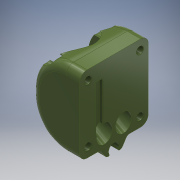
# Autodesk Inventor part: 3rd_phalanx_fingertip
Saved by Autodesk Inventor 2017 (Build 210142000, 142)
## iProperties
Created: 2017-06-28
Part Number: 3rd_phalanx_fingertip
Material: Generic
Document SubType Name: Modeling
Designer: Tomasz
Density: 1 g/cm^3
Appearance: Dark Olive
Author: Tomasz
Autodesk Inventor part; units mm, degrees
sketch "Sketch1" plane through (0, 0, 0) normal (0, 1, 0) x (-1, 0, 0)
  line L0 (0, 0) -> (1.5, 0)
  line L1 (1.5, -20) -> (0, -20)
  line L2 (0, -20) -> (0, 0)
  line L3 (1.5, 0) -> (3.5, 0)
  line L4 (12.5, -9) -> (12.5, -11)
  line L5 (3.5, -20) -> (1.5, -20)
  arc A0 (12.5, -9) -> (3.5, 0) centre (3.5, -9) ccw
  arc A1 (3.5, -20) -> (12.5, -11) centre (3.5, -11) ccw
  dimension "d0" = 20
  dimension "d4" = 9
  dimension "d5" = 12.5
  constraints: 12 end point, 4 point on circle, 4 tangent, 2 centre point, 2 horizontal, 2 parallel, 1 equal radius, 1 perpendicular, 1 point on line
  measures "d0" distance between parallel lines of L1 L0
  measures "d4" radius of A0
  measures "d5" distance between parallel lines of L4 L2
extrude "Extrusion1" add sketch "Sketch1" along normal blind 18
sketch "Sketch2" plane through (0, 0, 0) normal (1, 0, 0) x (0, 0, -1)
  line L0 (20, 0) -> (0, 0) projected
  line L1 (20, 0) -> (20, 18) projected
  line L2 (0, 18) -> (20, 18) projected
  line L3 (0, 0) -> (0, 18) projected
  line L4 (10, 0) -> (10, 18) construction
  line L5 (0, 0) -> (0, 18) projected
  line L6 (0, 9) -> (20, 9) construction
  point P0 (2.5, 2.2)
  point P1 (17.5, 2.2)
  point P2 (2.5, 15.8)
  point P3 (17.5, 15.8)
  dimension "d8" = 2.2
  dimension "d9" = 15
  constraints: 4 end point, 4 midpoint, 3 symmetric about line
  measures "d8" distance from line of L0 point (2.5, 2.2)
  measures "d9" distance of point (17.5, 2.2) point (2.5, 2.2)
hole "Hole1" at (0, 2.2, -2.5) at (0, 2.2, -17.5) at (0, 15.8, -2.5) at (0, 15.8, -17.5) direction (-1, 0, 0) diameter 1.9 end through all
ref_plane "Work Plane1" through (-2.5, 0, 0) normal (1, 0, 0) x (0, 0, -1)
sketch "Sketch3" plane through (-2.5, 0, 0) normal (1, 0, 0) x (0, 0, -1)
  spline S0 degree 2 poles (3.45, 2.2) (3.45, 0.5546) (2.025, 1.3773) (0.6, 2.2) (2.025, 3.0227) (3.45, 3.8454) (3.45, 2.2) knots 0 0 0 0.333333 0.333333 0.666667 0.666667 1 1 1 weights 1 0.5 1 0.5 1 0.5 1 projected
  spline S1 degree 2 poles (3.45, 15.8) (3.45, 14.1546) (2.025, 14.9773) (0.6, 15.8) (2.025, 16.6227) (3.45, 17.4454) (3.45, 15.8) knots 0 0 0 0.333333 0.333333 0.666667 0.666667 1 1 1 weights 1 0.5 1 0.5 1 0.5 1 projected
  spline S2 degree 2 poles (18.45, 15.8) (18.45, 14.1546) (17.025, 14.9773) (15.6, 15.8) (17.025, 16.6227) (18.45, 17.4454) (18.45, 15.8) knots 0 0 0 0.333333 0.333333 0.666667 0.666667 1 1 1 weights 1 0.5 1 0.5 1 0.5 1 projected
  spline S3 degree 2 poles (18.45, 2.2) (18.45, 0.5546) (17.025, 1.3773) (15.6, 2.2) (17.025, 3.0227) (18.45, 3.8454) (18.45, 2.2) knots 0 0 0 0.333333 0.333333 0.666667 0.666667 1 1 1 weights 1 0.5 1 0.5 1 0.5 1 projected
  circle A0 centre (2.5, 2.2) radius 0.95 projected
  circle A1 centre (2.5, 15.8) radius 0.95 projected
  circle A2 centre (17.5, 2.2) radius 0.95 projected
  circle A3 centre (17.5, 15.8) radius 0.95 projected
  circle A4 centre (2.5, 2.2) radius 1.75
  circle A5 centre (2.5, 15.8) radius 1.75
  circle A6 centre (17.5, 2.2) radius 1.75
  circle A7 centre (17.5, 15.8) radius 1.75
  point P0 (0, 0)
  dimension "d18" = 3.5
  dimension "d19" = 3.5
  dimension "d20" = 3.5
  dimension "d21" = 3.5
  constraints: 4 centre point, 4 coincident, 8 other
  measures "d18" diameter of A4
  measures "d19" diameter of A5
  measures "d20" diameter of A6
  measures "d21" diameter of A7
extrude "Extrusion2" cut sketch "Sketch3" against normal through all
sketch "Sketch4" plane through (0, 0, 0) normal (1, 0, 0) x (0, 0, -1)
  line L0 (4, 4.25) -> (16, 4.25)
  line L1 (16, 4.25) -> (16, 5.95)
  line L2 (16, 5.95) -> (4, 5.95)
  line L3 (4, 5.95) -> (4, 4.25)
  circle A0 centre (2.5, 15.8) radius 0.95 projected
  circle A1 centre (2.5, 2.2) radius 0.95 projected
  circle A2 centre (17.5, 2.2) radius 0.95 projected
  circle A3 centre (17.5, 15.8) radius 0.95 projected
  line L4 (20, 0) -> (0, 0) projected
  line L5 (20, 0) -> (20, 18) projected
  line L6 (0, 18) -> (20, 18) projected
  line L7 (0, 0) -> (0, 18) projected
  line L8 (0, 18) -> (20, 18) projected
  line L9 (20, 0) -> (0, 0) projected
  line L10 (10, 0) -> (10, 18) construction
  dimension "d25" = 12
  dimension "d26" = 1.7
  dimension "d29" = 4.25
  constraints: 10 end point, 2 midpoint, 2 parallel, 1 horizontal, 1 perpendicular, 1 other
  measures "d25" distance between parallel lines of L1 L3
  measures "d26" distance between parallel lines of L0 L2
  measures "d29" distance between parallel lines of L4 L0
extrude "Extrusion3" cut sketch "Sketch4" against normal blind 0.6 contours L3 L2 L1 L0
fillet "Fillet1" radius 2 10 edges at (-1.75, 0, -20) (-12.5, 0, -10) (-9.864, 0, -2.636) (-1.75, 0, 0) (-9.864, 0, -17.364) (-12.5, 18, -10) (-9.864, 18, -2.636) (-1.75, 18, 0) (-1.75, 18, -20) (-9.864, 18, -17.364)
ref_plane "Work Plane2" through (0, 9, 0) normal (0, -1, 0) x (1, 0, 0)
sketch "OptoForce_Offset" plane through (0, 9, 0) normal (0, -1, 0) x (1, 0, 0)
  line L0 (0, 0) -> (0, -20) projected
  line L1 (0, -10) -> (-16.7934, -10) construction
  point P0 (-10, -4)
  dimension "d30" = 10
  dimension "d31" = 6
  constraints: 2 end point, 1 horizontal, 1 midpoint
  measures "d30" distance from line of point (-10, -4) L0
  measures "d31" distance from line of point (-10, -4) L1
ref_plane "OptoForce_OffsetPlane" through (-10, 9, -4) normal (1, 0, 0) x (0, 0, -1)
sketch "OptoForce_RotationAxis" plane through (-10, 9, -4) normal (1, 0, 0) x (0, 0, -1)
  line L0 (0, 0) -> (0, 16)
  point P0 (-4, -9)
  constraints: 2 end point, 1 vertical
ref_plane "OptoForce_RotatedPlane" through (-10, 9, -4) normal (0.8660254, 0, -0.5) x (0, 1, 0)
sketch "OptoForce_SphereCenter" plane through (-10, 9, -4) normal (0.8660254, 0, -0.5) x (0, 1, 0)
  point P0 (-9, 8.4641)
  point P1 (0, 0)
ref_plane "OptoForce_OriginPlane" through (-5.6699, 9, -6.5) normal (0.8660254, 0, -0.5) x (0, 1, 0)
sketch "OptoForce_OriginSketch" plane through (-5.6699, 9, -6.5) normal (0.8660254, 0, -0.5) x (0, 1, 0)
  arc A0 (5.75, 0) -> (-5.75, 0) centre (0, 0) ccw
  line L0 (-5.75, 0) -> (-5.75, -4.25)
  line L1 (-0.5, -9.5) -> (0.5, -9.5)
  line L2 (5.75, -4.25) -> (5.75, 0)
  arc A1 (0.5, -9.5) -> (5.75, -4.25) centre (0.5, -4.25) ccw
  arc A2 (-5.75, -4.25) -> (-0.5, -9.5) centre (-0.5, -4.25) ccw
  point P0 (-9, 8.4641)
  dimension "d36" = 11.5
  dimension "d37" = 15.25
  dimension "d38" = 5.25
  constraints: 6 end point, 6 point on circle, 6 tangent, 3 centre point, 2 vertical, 1 coincident, 1 equal radius, 1 perpendicular
  measures "d36" diameter of A0
  measures "d38" radius of A1
extrude "Extrusion4" cut sketch "OptoForce_OriginSketch" against normal through all
sketch "Sketch11" plane through (-5.6699, 9, -6.5) normal (-0.8660254, 0, 0.5) x (0.5, 0, 0.8660254)
  arc A0 (0, -5.75) -> (0, 5.75) centre (0, 0) ccw projected
  line L0 (0, 5.75) -> (-4.25, 5.75) projected
  line L1 (-4.25, -5.75) -> (0, -5.75) projected
  line L2 (0, 0) -> (-14.8035, 0) construction
  line L3 (-6, -5) -> (-6, 4.6962) construction
  arc A1 (-9.5, -0.5) -> (-4.25, -5.75) centre (-4.25, -0.5) ccw projected
  arc A2 (-4.25, 5.75) -> (-9.5, 0.5) centre (-4.25, 0.5) ccw projected
  line L4 (-9.5, 0.5) -> (-9.5, -0.5) projected
  point P0 (8.4641, -9)
  point P1 (-6, -2.5)
  point P2 (-6, 2.5)
  dimension "d41" = 6
  dimension "d42" = 5
  constraints: 4 end point, 1 horizontal, 1 point on line, 1 symmetric about line, 1 vertical
  measures "d41" distance from line of L3 L2.start
  measures "d42" distance of point (-6, 2.5) point (-6, -2.5)
hole "Hole2" at (-8.6699, 6.5, -11.6962) at (-8.6699, 11.5, -11.6962) direction (0.8660254, 0, -0.5) diameter 2.4 end through all
sketch "Sketch12" plane through (-5.6699, 9, -6.5) normal (0.8660254, 0, -0.5) x (0, 1, 0)
  arc A0 (-3.5347, -5.3923) -> (-3.05, -4.9335) centre (-2.5, -6) ccw projected
  arc A1 (-3.05, -4.9335) -> (-3.6599, -5.6923) centre (-2.5, -6) ccw projected
  arc A2 (-3.5347, -5.3923) -> (-3.6599, -5.6923) centre (-2.5, -6) ccw projected
  circle A3 centre (-2.5, -6) radius 1.2 projected
  circle A4 centre (2.5, -6) radius 1.2 projected
  circle A5 centre (2.5, -6) radius 1.2 projected
  line L0 (-15, -8) -> (18.6629, -8)
  point P0 (-9, 8.4641)
  dimension "d51" = 2
  constraints: 2 end point, 1 horizontal
  measures "d51" distance from line of L0 A0.centre
ref_plane "Work Plane8" through (-9.6699, -6, -13.4282) normal (-0.5, 0, -0.8660254) x (0, 1, 0)
sketch "Sketch13" plane through (-9.6699, -6, -13.4282) normal (-0.5, 0, -0.8660254) x (0, 1, 0)
  ellipse E0 centre (12.5, 10.0111) end of major axis (13.7, 10.0111) minor radius 0.6928 (11.95, 9.3953) -> (11.4653, 9.6603) ccw projected
  line L0 (11.95, 8.7025) -> (11.95, 9.3953) projected
  ellipse E1 centre (12.5, 9.3183) end of major axis (13.7, 9.3183) minor radius 0.6928 (11.3401, 9.1406) -> (11.95, 8.7025) ccw projected
  ellipse E2 centre (12.5, 8.6077) end of major axis (12.5, 10.6862) minor radius 1.2 (11.4653, 9.6603) -> (11.3401, 9.1406) ccw projected
  line L1 (13.7, 0) -> (11.3, 0) construction
  ellipse E3 centre (17.5, 10.0111) end of major axis (18.7, 10.0111) minor radius 0.6928 projected
  line L2 (18.7, 0) -> (16.3, 0) projected
  line L3 (17.5, 0) -> (12.5, 0) construction
  line L4 (12.5, 0) -> (12.5, -4) construction
  line L5 (12.5, -4) -> (17.5, -4) construction
  line L6 (17.5, -4) -> (17.5, 0) construction
  line L7 (15, -4) -> (15, 0) construction
  arc A0 (17, -2) -> (13, -2) centre (15, -2) ccw
  line L8 (13, -2) -> (13, -6)
  line L9 (13, -6) -> (17, -6)
  line L10 (17, -6) -> (17, -2)
  point P0 (6, 1.6603)
  dimension "d53" = 4
  dimension "d54" = 4
  dimension "d55" = 2
  constraints: 16 end point, 5 midpoint, 2 horizontal, 2 parallel, 2 point on circle, 2 tangent, 2 vertical, 1 centre point, 1 perpendicular, 1 point on line, 4 other
  measures "d53" distance between parallel lines of L5 L3
  measures "d54" distance from line of L9 A0.centre
  measures "d55" radius of A0
extrude "Extrusion5" cut sketch "Sketch13" along normal through all contours L10 L9 L8 A0
ref_plane "Work Plane9" through (-4.3708, 9, -7.25) normal (0.8660254, 0, -0.5) x (0, 1, 0)
sketch "Sketch14" plane through (-4.3708, 9, -7.25) normal (0.8660254, 0, -0.5) x (0, 1, 0)
  arc A0 (-3.5347, -5.3923) -> (-3.05, -4.9335) centre (-2.5, -6) ccw projected
  arc A1 (-3.05, -4.9335) -> (-3.6599, -5.6923) centre (-2.5, -6) ccw projected
  arc A2 (-3.5347, -5.3923) -> (-3.6599, -5.6923) centre (-2.5, -6) ccw projected
  circle A3 centre (-2.5, -6) radius 1.2 projected
  circle A4 centre (2.5, -6) radius 1.2 projected
  circle A5 centre (2.5, -6) radius 1.2 projected
  circle A6 centre (-2.5, -6) radius 2.1
  circle A7 centre (2.5, -6) radius 2.1
  point P0 (-9, 8.4641)
  dimension "d59" = 4.2
  dimension "d60" = 4.2
  constraints: 2 centre point, 2 coincident
  measures "d59" diameter of A6
  measures "d60" diameter of A7
extrude "Extrusion6" cut sketch "Sketch14" along normal through all
sketch "Sketch15" plane through (0, 0, -2) normal (1, 0, 0) x (0, 0, -1)
  line L0 (-2, 2) -> (-2, 16) projected
  line L1 (-2, 9) -> (24.8317, 9) construction
  arc A0 (20.4, 9.9798) -> (18, 9) centre (19.4, 9) ccw
  line L2 (18, 2) -> (18, 16) projected
  line L3 (20.4, 11) -> (20.4, 9.9798)
  line L4 (20.4, 11) -> (18, 12.5)
  line L5 (18, 9) -> (18, 12.5)
  line L6 (18, 2) -> (18, 16) projected
  point P0 (-2, 0)
  dimension "d64" = 2.8
  dimension "d65" = 2
  dimension "d66" = 1
  dimension "d68" = 3.5
  constraints: 8 end point, 4 point on line, 3 midpoint, 2 point on circle, 1 centre point, 1 collinear, 1 horizontal, 1 parallel, 1 tangent
  measures "d64" diameter of A0
  measures "d65" distance from line of L4.start L1
  measures "d66" distance from line of L3 A0.centre
  measures "d68" distance of L5.start L4.end
extrude "Extrusion7" add sketch "Sketch15" against normal blind 3.5
fillet "Fillet2" radius 1 2 edges at (-1.75, 11, -22.4) (-1.75, 12.5, -20)
fillet "Fillet3" radius 0.2 1 edges at (-1.75, 9.9798, -22.4)
mirror "Mirror2" about plane through (0, 9, 0) normal (0, -1, 0) of "Fillet2", "Fillet3", "Extrusion7"
sketch "Sketch16" plane through (0, 16, -20) normal (0, 0, -1) x (-1, 0, 0)
  line L0 (0, -6.6) -> (0, -2.4) projected
  line L1 (0, -1.15) -> (0, 0.75) projected
  line L2 (3.5, -2.9458) -> (3.5, 0) projected
  line L3 (0, -1.15) -> (0, 0.75) projected
  line L4 (0, -1.15) -> (3.5, -1.15) construction
  line L5 (0, -2.4) -> (3.5, -2.4) construction
  line L6 (3.5, -1.775) -> (0, -1.775) construction
  line L7 (0, -2.9458) -> (0, 0) projected
  line L8 (0, -8.4) -> (0, -5.6) projected
  line L9 (0, -7) -> (8.9367, -7) construction
  point P0 (0, -16)
  point P1 (1.75, -1.775)
  point P2 (0, -8.2124)
  point P3 (0, -5.7876)
  point P4 (1.75, -12.225)
  constraints: 8 end point, 4 point on line, 2 horizontal, 2 midpoint, 1 parallel, 1 perpendicular, 1 symmetric about line, 1 other
hole "Hole3" at (-1.75, 14.225, -20) at (-1.75, 3.775, -20) direction (0, 0, 1) diameter 1.22 depth 2.2 tip angle 118
equation "\"d8\" = fingertip_mounting_dist_from_edge"
equation "\"d9\" = fingertip_mount_spacing"
equation "\"d19\" = d18"
equation "\"d20\" = d18"
equation "\"d21\" = d18"
equation "\"d30\" = OptoForce_Offset_Parallel"
equation "\"d31\" = OptoForce_Offset_Perpendicular"
equation "\"OptoForce_Offset_Perpendicular\" = 6"
equation "\"OptoForce_Offset_Parallel\" = 10"
equation "\"OptoForce_Angle\" = 30deg"
equation "\"d34\" = OptoForce_Angle"
equation "\"fingertip_mounting_dist_from_edge\" = 2.2"
equation "\"fingertip_mount_spacing\" = 15"
body "Solid1"
